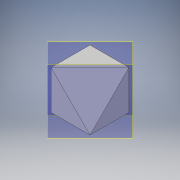
# Autodesk Inventor part: jimscube
Saved by Autodesk Inventor 2019 (Build 230136000, 136)
## iProperties
Created: 2019-09-15
Part Number: jimscube
Material: Generic
Document SubType Name: Modeling
Designer: james
Density: 1 g/cm^3
Appearance: Default
Author: james
Autodesk Inventor part; units mm, degrees
ref_plane "YZ Plane" through (0, 0, 0) normal (1, 0, 0) x (0, 1, 0)
ref_plane "XZ Plane" through (0, 0, 0) normal (0, 1, 0) x (-1, 0, 0)
ref_plane "XY Plane" through (0, 0, 0) normal (0, 0, 1) x (1, 0, 0)
sketch "Sketch1" plane through (0, 0, 0) normal (0, 1, 0) x (-1, 0, 0)
  line L0 (12.7, 12.7) -> (-12.7, 12.7)
  line L1 (-12.7, 12.7) -> (-12.7, -12.7)
  line L2 (-12.7, -12.7) -> (12.7, -12.7)
  line L3 (12.7, -12.7) -> (12.7, 12.7)
  point P0 (0, 0)
  dimension "d0" = 12.7
  dimension "d1" = 25.4
  dimension "d2" = 25.4
  dimension "d3" = 12.7
  constraints: 8 end point, 2 parallel, 1 horizontal, 1 perpendicular
  measures "d0" distance from line of L2 point (0, 0)
  measures "d1" distance of L2.end L0.start
  measures "d2" distance of L0.start L0.end
  measures "d3" distance from line of point (0, 0) L3
extrude "Extrusion1" add sketch "Sketch1" along normal blind 25.4
ref_plane "Work Plane1" through (-12.7, 25.4, 12.7) normal (-0.5773503, -0.5773503, -0.5773503) x (0.7071068, 0, -0.7071068)
sketch "Sketch2" plane through (-12.7, 25.4, 12.7) normal (-0.5773503, -0.5773503, -0.5773503) x (0.7071068, 0, -0.7071068)
  line L0 (-1.8052, -5.2104) -> (39.1986, -5.2104)
  line L1 (39.1986, -5.2104) -> (39.1986, 33.6585)
  line L2 (39.1986, 33.6585) -> (-1.8052, 33.6585)
  line L3 (-1.8052, 33.6585) -> (-1.8052, -5.2104)
  point P0 (17.9605, 20.739)
  constraints: 8 end point, 2 parallel, 1 horizontal, 1 perpendicular
extrude "Extrusion2" cut sketch "Sketch2" against normal blind 25.4
ref_plane "Work Plane2" through (12.7, 0, -12.7) normal (-0.5773503, -0.5773503, -0.5773503) x (-0.7071068, 0, 0.7071068)
sketch "Sketch3" plane through (12.7, 0, -12.7) normal (-0.5773503, -0.5773503, -0.5773503) x (-0.7071068, 0, 0.7071068)
  line L0 (-4.9386, 41.2898) -> (46.8411, 41.2898)
  line L1 (46.8411, 41.2898) -> (46.8411, -12.9896)
  line L2 (46.8411, -12.9896) -> (-4.9386, -12.9896)
  line L3 (-4.9386, -12.9896) -> (-4.9386, 41.2898)
  point P0 (17.9605, 0)
  constraints: 8 end point, 2 parallel, 1 horizontal, 1 perpendicular
extrude "Extrusion3" cut sketch "Sketch3" along normal blind 25.4
body "Solid1"
